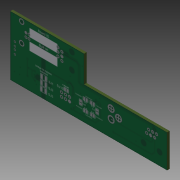
# Autodesk Inventor part: pcb
Saved by Autodesk Inventor 2014 SP1 (Build 180222100, 222)
## iProperties
Created: 2014-04-06
Part Number: pcb
Material: Generic
Document SubType Name: Modeling
Designer: Tyler
Density: 1 g/cm^3
Appearance: Default
Author: Tyler
Autodesk Inventor part; units mm, degrees
ref_plane "YZ Plane" through (0, 0, 0) normal (1, 0, 0) x (0, 1, 0)
ref_plane "XZ Plane" through (0, 0, 0) normal (0, 1, 0) x (-1, 0, 0)
ref_plane "XY Plane" through (0, 0, 0) normal (0, 0, 1) x (1, 0, 0)
sketch "Sketch1" plane through (0, 0, 0) normal (0, 1, 0) x (-1, 0, 0)
  line L0 (-50, 10.5) -> (3, 10.5)
  line L1 (50, -2.7166) -> (50, -10.5)
  line L2 (50, -10.5) -> (-50, -10.5)
  line L3 (-50, -10.5) -> (-50, 10.5)
  line L4 (50, -2.7166) -> (50, 27.5)
  line L5 (50, 27.5) -> (3, 27.5)
  line L6 (3, 27.5) -> (3, 10.5)
  point P0 (0, 0)
  dimension "d0" = 47
  dimension "d1" = 17
  dimension "d2" = 100
  dimension "d3" = 21
  dimension "d4" = 10.5
  dimension "d5" = 50
  constraints: 14 end point, 4 parallel, 2 perpendicular, 1 horizontal
  measures "d0" distance of L4.end L5.end
  measures "d1" distance between parallel lines of L0 L5
  measures "d2" distance between parallel lines of L3 L1
  measures "d3" distance between parallel lines of L0 L2
  measures "d4" distance from line of point (0, 0) L0
  measures "d5" distance from line of point (0, 0) L3
extrude "Extrusion1" add sketch "Sketch1" along normal blind 1.6
equation "\"d4\" = 0.5 * d3"
equation "\"d5\" = 0.5 * d2"
body "Solid1"
